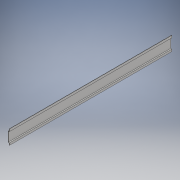
# Autodesk Inventor part: Koffer_ankerschiene_15m
Saved by Autodesk Inventor 2018 (Build 220112000, 112)
## iProperties
Created: 2020-03-29
Part Number: Koffer_ankerschiene_15m
Material: Generisch
Document SubType Name: Blech
Designer: wepet
Density: 1 g/cm^3
Sheet Metal Rule: Standard_mm
Appearance: Vorgabe
Author: wepet
Autodesk Inventor part; units mm, degrees
ref_plane "YZ Plane" through (0, 0, 0) normal (1, 0, 0) x (0, 1, 0)
ref_plane "XZ Plane" through (0, 0, 0) normal (0, 1, 0) x (-1, 0, 0)
ref_plane "XY Plane" through (0, 0, 0) normal (0, 0, 1) x (1, 0, 0)
sketch "Skizze1" plane through (0, 0, 0) normal (0, 1, 0) x (-1, 0, 0)
  line L0 (0, 0) -> (1.15, 0) construction
  line L1 (1.15, 0) -> (1.15, -13) construction
  line L2 (1.15, -13) -> (0, -13) construction
  line L3 (0, -13) -> (0, 0) construction
  line L4 (0, -6.5) -> (1.15, -6.5) construction
  line L5 (0.575, -1.85) -> (0.575, -11.15) construction
  line L6 (0.3, -1.7763) -> (1.15, -2.0041) construction
  line L7 (0.85, -2.2343) -> (0, -2.0065) construction
  line L8 (0.3, 0) -> (0.3, -1.7763)
  line L9 (0.3, -11.2237) -> (1.15, -10.9959) construction
  line L10 (0, -10.9935) -> (0.85, -10.7657) construction
  line L11 (0.3, -11.2237) -> (0.3, -13)
  line L12 (0.85, -2.2343) -> (0.85, -10.7657)
  line L13 (0, 0) -> (0.3, 0)
  line L14 (0.3, -1.7763) -> (1.15, -2.0041)
  line L15 (1.15, -10.9959) -> (0.3, -11.2237)
  line L16 (0.3, -13) -> (0, -13)
  line L17 (0, -10.9935) -> (0.85, -10.7657)
  line L18 (0.85, -2.2343) -> (0, -2.0065)
  line L19 (1.15, -2.0041) -> (1.15, -10.9959)
  line L20 (0, -2.0065) -> (0, 0)
  line L21 (0, -10.9935) -> (0, -13)
  point P0 (0.575, -6.5)
  dimension "d0" = 1.15
  dimension "d1" = 13
  dimension "d4" = 9.3
  dimension "d7" = 75
  dimension "d8" = 0.3
  dimension "d9" = 0.3
  dimension "d10" = 75
  dimension "d11" = 0.3
  dimension "d12" = 0.3
  constraints: 44 end point, 8 point on line, 7 collinear, 7 parallel, 5 perpendicular, 4 midpoint, 1 horizontal
  measures "d0" distance of L1.end L2.end
  measures "d1" distance of L0.end L1.end
  measures "d4" distance of L5.end L5.start
  measures "d7" angle of L6 L3
  measures "d8" distance between parallel lines of L7 L6
  measures "d9" distance between parallel lines of L3 L8
  measures "d10" angle of L3 L9
  measures "d11" distance between parallel lines of L9 L10
  measures "d12" distance between parallel lines of L1 L12
extrude "Extrusion1" add sketch "Skizze1" along normal blind 150
equation "\"Biegeradius\" = Stärke"
equation "\"BreiteBiegungsfreistellung\" = Stärke"
equation "\"TiefeBiegungsfreistellung\" = 0.5 * Stärke"
equation "\"GrößeEckenfreistellung\" = 4 * Stärke"
equation "\"MinimalRest\" = 2 * Stärke"
equation "\"Übergangsradius\" = Biegeradius"
equation "\"JacobiRadiusGröße\" = Biegeradius"
equation "\"Abstandsgröße\" = Stärke"
equation "\"Stärke\" = 0.5"
